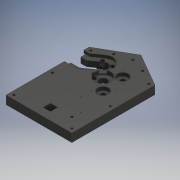
# Autodesk Inventor part: AC02
Saved by Autodesk Inventor 2017 (Build 210142000, 142)
## iProperties
Created: 2019-08-28
Part Number: AC02
Material: ABS Plastic
Document SubType Name: Modeling
Designer: Dell
Density: 1.06 g/cm^3
Appearance: Smooth - Black
Author: Dell
Autodesk Inventor part; units mm, degrees
ref_plane "YZ Plane" through (0, 0, 0) normal (1, 0, 0) x (0, 1, 0)
ref_plane "XZ Plane" through (0, 0, 0) normal (0, 1, 0) x (-1, 0, 0)
ref_plane "XY Plane" through (0, 0, 0) normal (0, 0, 1) x (1, 0, 0)
sketch "Sketch35" plane through (0, 0, 0) normal (0, 0, 1) x (1, 0, 0)
  line L0 (0, 68.1273) -> (59, 34.0637)
  line L1 (59, 34.0637) -> (59, -34.0637)
  line L2 (59, -34.0637) -> (0, -68.1273)
  line L3 (0, -68.1273) -> (-59, -34.0637)
  line L4 (-59, -34.0637) -> (-59, 34.0637)
  line L5 (-59, 34.0637) -> (0, 68.1273)
  line L6 (-59, -34.0637) -> (-59, -115)
  line L7 (-59, -115) -> (59, -115)
  line L8 (59, -115) -> (59, -34.0637)
  point P0 (0, 0)
  point P1 (0, 0)
  dimension "d165" = 118
  dimension "d166" = 115
  constraints: 18 end point, 2 perpendicular, 1 coincident, 1 vertical, 1 vertical alignment, 13 other
  measures "d165" distance between parallel lines of L1 L4
  measures "d166" distance from line of L7 point (0, 0)
extrude "Extrusion34" add sketch "Sketch35" along normal blind 55
sketch "Sketch36" plane through (0, 0, 55) normal (0, 0, 1) x (1, 0, 0)
  line L0 (59, -115) -> (59, 34.0637) construction
  line L1 (59, 34.0637) -> (0, 68.1273) construction
  line L2 (0, 68.1273) -> (-59, 34.0637) construction
  line L3 (-59, 34.0637) -> (-59, -115) construction
  line L4 (-59, -115) -> (59, -115) construction
  line L5 (52, 30.0222) -> (52, -108) construction
  line L6 (52, -108) -> (-52, -108) construction
  line L7 (-52, -108) -> (-52, 30.0222) construction
  line L8 (-52, 30.0222) -> (0, 60.0444) construction
  line L9 (0, 60.0444) -> (52, 30.0222) construction
  circle A0 centre (-52, -108) radius 2
  circle A1 centre (52, -108) radius 2
  circle A2 centre (0, 60.0444) radius 2
  circle A3 centre (-52, 30.0222) radius 2
  circle A4 centre (52, 30.0222) radius 2
  circle A5 centre (-26, -108) radius 2
  circle A6 centre (26, -108) radius 2
  circle A7 centre (0, -108) radius 2
  circle A8 centre (-52, -68.9889) radius 2
  circle A9 centre (-52, -38.9889) radius 2
  circle A10 centre (-52, 0) radius 2
  circle A11 centre (52, 0) radius 2
  circle A12 centre (52, -38.9889) radius 2
  circle A13 centre (52, -68.9889) radius 2
  circle A14 centre (-26, 45.0333) radius 2
  circle A15 centre (26, 45.0333) radius 2
  point P0 (0, 0)
  dimension "d169" = 7
  dimension "d170" = 4
  dimension "d171" = 4
  dimension "d172" = 4
  dimension "d173" = 4
  dimension "d174" = 4
  dimension "d175" = 4
  dimension "d176" = 4
  dimension "d177" = 4
  dimension "d178" = 4
  dimension "d179" = 4
  dimension "d180" = 4
  dimension "d181" = 4
  dimension "d182" = 4
  dimension "d183" = 4
  dimension "d184" = 4
  dimension "d185" = 4
  dimension "d186" = 30
  constraints: 16 centre point, 10 end point, 6 point on line, 5 coincident, 5 midpoint, 3 horizontal alignment, 2 vertical alignment, 4 other
  measures "d169" distance between parallel lines of L0 L5
  measures "d170" diameter of A0
  measures "d171" diameter of A1
  measures "d172" diameter of A2
  measures "d173" diameter of A3
  measures "d174" diameter of A4
  measures "d175" diameter of A5
  measures "d176" diameter of A6
  measures "d177" diameter of A7
  measures "d178" diameter of A8
  measures "d179" diameter of A9
  measures "d180" diameter of A10
  measures "d181" diameter of A11
  measures "d182" diameter of A12
  measures "d183" diameter of A13
  measures "d184" diameter of A14
  measures "d185" diameter of A15
  measures "d186" distance of A9.centre A8.centre
extrude "Extrusion35" cut sketch "Sketch36" against normal through all contours A0 | A1 | A3 | A4 | A9 | A12 | A14 | A15
sketch "Sketch37" plane through (0, 0, 55) normal (0, 0, 1) x (1, 0, 0)
  circle A0 centre (0, 0) radius 15
  dimension "d189" = 30
  constraints: 1 centre point, 1 coincident
  measures "d189" diameter of A0
extrude "Extrusion36" cut sketch "Sketch37" against normal blind 7
sketch "Sketch41" plane through (0, 0, 0) normal (0, 0, -1) x (-1, 0, 0)
  circle A0 centre (26, 45.0333) radius 2 projected
  circle A1 centre (-52, -38.9889) radius 2 projected
  circle A2 centre (-52, 30.0222) radius 2 projected
  circle A3 centre (52, -108) radius 2 projected
  circle A4 centre (-52, -108) radius 2 projected
  circle A5 centre (52, 30.0222) radius 2 projected
  circle A6 centre (52, -38.9889) radius 2 projected
  circle A7 centre (-26, 45.0333) radius 2 projected
  line L0 (-59, -115) -> (-59, 34.0637) projected
  line L1 (59, -115) -> (-59, -115) projected
  line L2 (59, 34.0637) -> (59, -115) projected
  line L3 (0, 68.1273) -> (59, 34.0637) projected
  line L4 (-59, 34.0637) -> (0, 68.1273) projected
  line L5 (0, 51.9615) -> (45, 25.9808)
  line L6 (45, 25.9808) -> (45, -101)
  line L7 (45, -101) -> (-45, -101)
  line L8 (-45, -101) -> (-45, 25.9808)
  line L9 (-45, 25.9808) -> (0, 51.9615)
  point P0 (0, 0)
  dimension "d199" = 14
  constraints: 10 end point, 4 other
  measures "d199" distance between parallel lines of L8 L0
extrude "Extrusion39" cut sketch "Sketch41" against normal blind 40 contours L0 L4 L3 L2 L1 | L5 L6 L7 L8 L9
sketch "Sketch42" plane through (0, 0, 40) normal (0, 0, -1) x (-1, 0, 0)
  circle A0 centre (0, 0) radius 7.5
  circle A1 centre (-21.9203, -21.9203) radius 4
  circle A2 centre (-17.6777, 17.6777) radius 4
  circle A3 centre (21.9203, 21.9203) radius 4
  line L0 (0, 0) -> (32.276, 0) construction
  line L1 (0, 0) -> (-21.9203, -21.9203) construction
  line L2 (0, 0) -> (-17.6777, 17.6777) construction
  line L3 (0, 0) -> (21.9203, 21.9203) construction
  line L4 (12.9203, 29.9203) -> (30.9203, 29.9203) construction
  line L5 (30.9203, 29.9203) -> (30.9203, -3.0797) construction
  line L6 (30.9203, -3.0797) -> (12.9203, -3.0797) construction
  line L7 (12.9203, -3.0797) -> (12.9203, 29.9203) construction
  circle A4 centre (12.9203, 29.9203) radius 1.75
  circle A5 centre (30.9203, 29.9203) radius 1.75
  circle A6 centre (30.9203, -3.0797) radius 1.75
  circle A7 centre (12.9203, -3.0797) radius 1.75
  point P0 (21.9203, 29.9203)
  dimension "d202" = 15
  dimension "d203" = 8
  dimension "d204" = 8
  dimension "d205" = 8
  dimension "d206" = 31
  dimension "d207" = 25
  dimension "d208" = 31
  dimension "d209" = 45
  dimension "d210" = 18
  dimension "d211" = 33
  dimension "d212" = 8
  dimension "d213" = 3.5
  dimension "d214" = 3.5
  dimension "d215" = 3.5
  dimension "d216" = 3.5
  dimension "d219" = 135
  dimension "d220" = 135
  constraints: 16 end point, 8 centre point, 5 coincident, 2 horizontal, 2 parallel, 1 midpoint, 1 perpendicular, 1 vertical alignment
  measures "d202" diameter of A0
  measures "d203" diameter of A1
  measures "d204" diameter of A2
  measures "d205" diameter of A3
  measures "d206" distance of point (0, 0) L3.end
  measures "d207" distance of point (0, 0) L2.end
  measures "d208" distance of point (0, 0) L1.end
  measures "d209" angle of L0 L3
  measures "d210" distance of L4.start L4.end
  measures "d211" distance of L4.end L5.end
  measures "d212" distance from line of L4 L3.end
  measures "d213" diameter of A4
  measures "d214" diameter of A5
  measures "d215" diameter of A6
  measures "d216" diameter of A7
  measures "d219" angle of L0 L1
  measures "d220" angle of L2 L0
extrude "Extrusion40" cut sketch "Sketch42" against normal through all
sketch "Sketch43" plane through (0, 0, 40) normal (0, 0, -1) x (-1, 0, 0)
  line L0 (-6.5, -88) -> (6.5, -88)
  line L1 (6.5, -88) -> (6.5, -101)
  line L2 (6.5, -101) -> (-6.5, -101)
  line L3 (-6.5, -101) -> (-6.5, -88)
  line L4 (59, -115) -> (-59, -115) projected
  point P0 (0, 0)
  point P1 (0, -88)
  dimension "d221" = 13
  dimension "d222" = 13
  dimension "d223" = 27
  constraints: 8 end point, 2 parallel, 1 horizontal, 1 midpoint, 1 perpendicular, 1 vertical alignment
  measures "d221" distance of L1.end L2.end
  measures "d222" distance of L0.end L1.end
  measures "d223" distance between parallel lines of L4 L0
extrude "Extrusion41" cut sketch "Sketch43" against normal through all
sketch "Sketch44" plane through (0, 0, 40) normal (0, 0, -1) x (-1, 0, 0)
  circle A0 centre (0, 53.1273) radius 2
  circle A1 centre (-34, -90) radius 2
  line L0 (-59, -115) -> (-59, 34.0637) projected
  line L1 (59, -115) -> (-59, -115) projected
  point P0 (0, 0)
  point P1 (0, 68.1273)
  dimension "d226" = 4
  dimension "d227" = 4
  dimension "d228" = 15
  dimension "d229" = 25
  dimension "d230" = 25
  constraints: 2 centre point, 1 vertical alignment
  measures "d226" diameter of A0
  measures "d227" diameter of A1
  measures "d228" distance of point (0, 68.127) A0.centre
  measures "d229" distance from line of L0 A1.centre
  measures "d230" distance from line of L1 A1.centre
extrude "Extrusion42" cut sketch "Sketch44" against normal through all
sketch "Sketch45" plane through (0, 0, 40) normal (0, 0, -1) x (-1, 0, 0)
  circle A0 centre (21.9203, 21.9203) radius 4 projected
  circle A1 centre (12.9203, 29.9203) radius 1.75 projected
  circle A2 centre (30.9203, 29.9203) radius 1.75 projected
  circle A3 centre (30.9203, -3.0797) radius 1.75 projected
  circle A4 centre (12.9203, -3.0797) radius 1.75 projected
  circle A5 centre (12.9203, -3.0797) radius 4.5
  circle A6 centre (12.9203, 29.9203) radius 7.5
  circle A7 centre (21.9203, 21.9203) radius 9
  circle A8 centre (30.9203, 29.9203) radius 1.75 projected
  circle A9 centre (30.9203, 29.9203) radius 7.5
  circle A10 centre (30.9203, -3.0797) radius 7.5
  point P0 (0, 0)
  dimension "d233" = 9
  dimension "d234" = 15
  dimension "d235" = 18
  dimension "d236" = 15
  dimension "d237" = 15
  constraints: 5 centre point, 5 coincident
  measures "d233" diameter of A5
  measures "d234" diameter of A6
  measures "d235" diameter of A7
  measures "d236" diameter of A9
  measures "d237" diameter of A10
extrude "Extrusion43" add sketch "Sketch45" along normal blind 2
sketch "Sketch47" plane through (0, 0, 55) normal (0, 0, 1) x (1, 0, 0)
  circle A0 centre (-21.9203, 21.9203) radius 4 projected
  circle A1 centre (-21.9203, 21.9203) radius 9
  line L0 (-27.0825, 29.2927) -> (-45.9755, 16.0637)
  line L1 (-45.9755, 16.0637) -> (-59, 16.0637)
  line L2 (-59, 34.0637) -> (-59, -115) projected
  line L3 (-59, 16.0637) -> (-59, -1.9363)
  line L4 (-59, -1.9363) -> (-40.3001, -1.9363)
  line L5 (-40.3001, -1.9363) -> (-16.7581, 14.5479)
  point P0 (0, 0)
  dimension "d242" = 18
  dimension "d243" = 18
  dimension "d244" = 145
  dimension "d245" = 18
  constraints: 10 end point, 2 horizontal, 2 point on circle, 2 point on line, 2 tangent, 1 centre point, 1 coincident, 1 parallel
  measures "d242" diameter of A1
  measures "d243" distance between parallel lines of L1 L4
  measures "d244" angle of L0 L1
  measures "d245" distance from line of L2.start L1
extrude "Extrusion45" cut sketch "Sketch47" against normal through all
fillet "Fillet1" radius 5 1 edges at (-45.9755, 16.0637, 47.5)
sketch "Sketch49" plane through (0, 0, 55) normal (0, 0, 1) x (1, 0, 0)
  circle A0 centre (-30.9203, 29.9203) radius 3.5
  circle A1 centre (-12.9203, 29.9203) radius 3.5
  circle A2 centre (-12.9203, -3.0797) radius 3.5
  circle A3 centre (-30.9203, -3.0797) radius 3.5
  circle A4 centre (-30.9203, 29.9203) radius 1.75 projected
  circle A5 centre (-30.9203, -3.0797) radius 1.75 projected
  arc A6 (-14.5047, -3.8228) -> (-14.6696, -3.1312) centre (-12.9203, -3.0797) ccw projected
  circle A7 centre (-12.9203, 29.9203) radius 1.75 projected
  point P0 (0, 0)
  dimension "d249" = 7
  dimension "d250" = 7
  dimension "d251" = 7
  dimension "d252" = 7
  constraints: 4 centre point, 4 coincident
  measures "d249" diameter of A0
  measures "d250" diameter of A1
  measures "d251" diameter of A2
  measures "d252" diameter of A3
extrude "Extrusion46" cut sketch "Sketch49" against normal blind 12 contours A0 | A1 | A2 | A3 | A4 | A5 | A7
sketch "Sketch50" plane through (0, 0, 55) normal (0, 0, 1) x (1, 0, 0)
  arc A0 (-16.2779, 28.9319) -> (-27.0825, 29.2927) centre (-21.9203, 21.9203) ccw projected
  circle A1 centre (-21.9203, 21.9203) radius 17.5
  line L0 (-31.9579, 36.2555) -> (-48.6555, 24.5637)
  line L1 (-48.6555, 24.5637) -> (-59, 24.5637)
  line L2 (-11.8827, 7.5851) -> (-37.6201, -10.4363)
  line L3 (-37.6201, -10.4363) -> (-59, -10.4363)
  line L4 (-59, -1.9363) -> (-59, -115) projected
  line L5 (-59, -10.4363) -> (-59, 24.5637)
  line L6 (-44.6841, 16.9679) -> (-31.1718, 26.4294) projected
  line L7 (-16.7581, 14.5479) -> (-40.3001, -1.9363) projected
  line L8 (-40.3001, -1.9363) -> (-59, -1.9363) projected
  line L9 (-59, 16.0637) -> (-47.552, 16.0637) projected
  line L10 (-59, 16.0637) -> (-59, -1.9363)
  point P0 (0, 0)
  point P1 (-59, 7.0637)
  dimension "d255" = 35
  dimension "d258" = 35
  constraints: 12 end point, 4 parallel, 2 horizontal, 2 midpoint, 2 point on circle, 2 tangent, 1 centre point, 1 coincident, 1 collinear, 1 point on line, 1 vertical
  measures "d255" diameter of A1
  measures "d258" distance between parallel lines of L3 L1
extrude "Extrusion47" cut sketch "Sketch50" against normal blind 5
sketch "Sketch52" plane through (-59, 34.0637, 40) normal (-1, 0, 0) x (0, 0, 1)
  line L0 (3, -7.6343) -> (10, -7.6343) projected
  line L1 (0, -149.0637) -> (0, 0) projected
  line L2 (10, -7.6343) -> (0, -7.6343)
  line L3 (0, -7.6343) -> (0, -44.5)
  line L4 (0, -44.5) -> (10, -44.5)
  line L5 (10, -44.5) -> (10, -7.6343)
  point P0 (-40, -34.0637)
  point P1 (10, -44.5)
  constraints: 8 end point, 2 parallel, 1 coincident, 1 horizontal, 1 perpendicular, 1 point on line
extrude "Extrusion48" cut sketch "Sketch52" against normal blind 3
sketch "Sketch53" plane through (0, 0, 55) normal (0, 0, 1) x (1, 0, 0)
  circle A0 centre (17.6777, 17.6777) radius 4 projected
  circle A1 centre (17.6777, 17.6777) radius 10
  circle A2 centre (21.9203, -21.9203) radius 4 projected
  circle A3 centre (21.9203, -21.9203) radius 10
  point P0 (0, 0)
  dimension "d261" = 20
  dimension "d262" = 20
  constraints: 2 centre point, 2 coincident
  measures "d261" diameter of A1
  measures "d262" diameter of A3
extrude "Extrusion49" cut sketch "Sketch53" against normal blind 6
sketch "Sketch54" plane through (0, 0, 40) normal (0, 0, -1) x (-1, 0, 0)
  circle A0 centre (-17.6777, 17.6777) radius 4 projected
  circle A1 centre (-17.6777, 17.6777) radius 10
  circle A2 centre (-21.9203, -21.9203) radius 4 projected
  circle A3 centre (-21.9203, -21.9203) radius 10
  point P0 (0, 0)
  dimension "d265" = 20
  dimension "d266" = 20
  constraints: 2 centre point, 2 coincident
  measures "d265" diameter of A1
  measures "d266" diameter of A3
extrude "Extrusion50" cut sketch "Sketch54" against normal blind 6
sketch "Sketch56" plane through (0, 0, 40) normal (0, 0, -1) x (-1, 0, 0)
  line L0 (-28.2843, 7.0711) -> (-7.0711, 28.2843) construction
  line L1 (0, 0) -> (-17.6777, 17.6777) construction
  circle A0 centre (-21.9203, -21.9203) radius 4 construction
  line L2 (0, 0) -> (-21.9203, -21.9203) construction
  line L3 (-32.5269, -11.3137) -> (-11.3137, -32.5269) construction
  circle A1 centre (-17.6777, 17.6777) radius 4 construction
  circle A2 centre (-7.0711, 28.2843) radius 0.75
  circle A3 centre (-28.2843, 7.0711) radius 0.75
  circle A4 centre (-32.5269, -11.3137) radius 0.75
  circle A5 centre (-11.3137, -32.5269) radius 0.75
  dimension "d272" = 30
  dimension "d273" = 30
  dimension "d274" = 1.5
  dimension "d275" = 1.5
  dimension "d276" = 1.5
  dimension "d277" = 1.5
  constraints: 8 end point, 5 coincident, 4 centre point, 2 midpoint, 2 perpendicular
  measures "d272" distance of L0.start L0.end
  measures "d273" distance of L3.start L3.end
  measures "d274" diameter of A2
  measures "d275" diameter of A3
  measures "d276" diameter of A4
  measures "d277" diameter of A5
extrude "Extrusion51" cut sketch "Sketch56" against normal through all
sketch "Sketch58" plane through (0, 0, 40) normal (0, 0, -1) x (-1, 0, 0)
  circle A0 centre (-35, -75) radius 0.75
  circle A1 centre (-10, -50) radius 0.75
  point P0 (0, 0)
  dimension "d286" = 1.5
  dimension "d287" = 1.5
  dimension "d288" = 50
  dimension "d289" = 10
  dimension "d290" = 25
  dimension "d291" = 25
  constraints: 2 centre point
  measures "d286" diameter of A0
  measures "d287" diameter of A1
  measures "d288" vertical distance of point (0, 0) A1.centre
  measures "d289" horizontal distance of A1.centre point (0, 0)
  measures "d290" horizontal distance of A1.centre A0.centre
  measures "d291" horizontal distance of A1.centre A0.centre
extrude "Extrusion53" cut sketch "Sketch58" against normal through all
equation "\"d213\" = d215"
equation "\"d214\" = d215"
equation "\"d216\" = d215"
equation "\"d243\" = d242"
equation "\"d258\" = d255"
body "Solid2"
